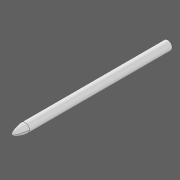
# Autodesk Inventor part: SealantApplicator
Saved by Autodesk Inventor 2020 (Build 240168000, 168)
## iProperties
Created: 2020-01-15
Part Number: SealantApplicator
Material: Generic
Document SubType Name: Modeling
Designer: Isaac Newcomb
Density: 1 g/cm^3
Appearance: Default
Author: Isaac Newcomb
Autodesk Inventor part; units mm, degrees
ref_plane "YZ Plane" through (0, 0, 0) normal (1, 0, 0) x (0, 1, 0)
ref_plane "XZ Plane" through (0, 0, 0) normal (0, 1, 0) x (-1, 0, 0)
ref_plane "XY Plane" through (0, 0, 0) normal (0, 0, 1) x (1, 0, 0)
sketch "Sketch1" plane through (0, 0, 0) normal (0, 1, 0) x (-1, 0, 0)
  line L0 (-5, -15) -> (-5, -180)
  line L1 (-5, -180) -> (0, -180)
  line L2 (0, -180) -> (0, 0)
  line L3 (0, 0) -> (-2, 0) construction
  line L4 (-2, 0) -> (-5, -10) construction
  line L5 (-5, -10) -> (-5, -15) construction
  spline S0 degree 3 poles (0, 0) (-2, 0) (-5, -10) (-5, -15) knots 1 1 1 1 2 2 2 2
  dimension "d1" = 5
  dimension "d2" = 15
  dimension "d3" = 5
  dimension "d4" = 2
  dimension "d5" = 180
  constraints: 6 end point, 2 perpendicular, 2 vertical, 1 horizontal, 3 other
  measures "d1" distance of L0.end L1.end
  measures "d2" vertical distance of L2.end L0.start
  measures "d3" distance of L4.end L0.start
  measures "d4" distance of L2.end L3.end
  measures "d5" distance of L1.end L2.end
revolve "Revolution1" add sketch "Sketch1" angle 360 about axis through (0, 0, -180) along (0, 0, 1)
body "Solid1"
